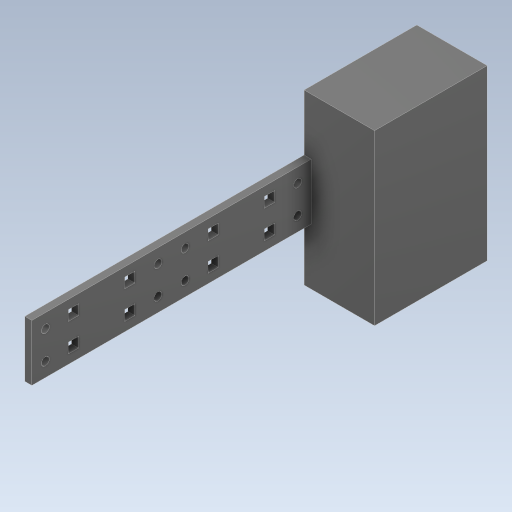
# Autodesk Inventor part: blocker
Saved by Autodesk Inventor 2024 (Build 280153000, 153)
## iProperties
Created: 2024-11-10
Part Number: blocker
Material: ABS Plastic
Document SubType Name: Modeling
Designer: Oscar
Density: 1.06 g/cm^3
Appearance: Smooth - Black
Author: Oscar
Autodesk Inventor part; units mm, degrees
ref_plane "YZ Plane" through (0, 0, 0) normal (1, 0, 0) x (0, 1, 0)
ref_plane "XZ Plane" through (0, 0, 0) normal (0, 1, 0) x (-1, 0, 0)
ref_plane "XY Plane" through (0, 0, 0) normal (0, 0, 1) x (1, 0, 0)
sketch "Sketch1" plane through (0, 0, 0) normal (1, 0, 0) x (0, 1, 0)
  line L0 (0, 0) -> (25.4, 0)
  line L1 (25.4, 0) -> (25.4, -126)
  line L2 (25.4, -126) -> (0, -126)
  line L3 (0, -126) -> (0, 0)
  line L4 (50.8, -126) -> (-25.4, -126)
  line L5 (-25.4, -126) -> (-25.4, -176.8)
  line L6 (-25.4, -176.8) -> (50.8, -176.8)
  line L7 (50.8, -176.8) -> (50.8, -126)
  line L8 (8.6614, -41.8886) -> (4.0386, -41.8886)
  line L9 (4.0386, -41.8886) -> (4.0386, -46.5114)
  line L10 (4.0386, -46.5114) -> (8.6614, -46.5114)
  line L11 (8.6614, -46.5114) -> (8.6614, -41.8886)
  line L12 (8.6614, -16.4886) -> (4.0386, -16.4886)
  line L13 (4.0386, -16.4886) -> (4.0386, -21.1114)
  line L14 (4.0386, -21.1114) -> (8.6614, -21.1114)
  line L15 (8.6614, -21.1114) -> (8.6614, -16.4886)
  line L16 (21.3614, -41.8886) -> (16.7386, -41.8886)
  line L17 (16.7386, -41.8886) -> (16.7386, -46.5114)
  line L18 (16.7386, -46.5114) -> (21.3614, -46.5114)
  line L19 (21.3614, -46.5114) -> (21.3614, -41.8886)
  line L20 (21.3614, -16.4886) -> (16.7386, -16.4886)
  line L21 (16.7386, -16.4886) -> (16.7386, -21.1114)
  line L22 (16.7386, -21.1114) -> (21.3614, -21.1114)
  line L23 (21.3614, -21.1114) -> (21.3614, -16.4886)
  line L24 (25.4, -63) -> (0, -63) construction
  line L25 (8.6614, -84.1114) -> (4.0386, -84.1114)
  line L26 (4.0386, -84.1114) -> (4.0386, -79.4886)
  line L27 (4.0386, -79.4886) -> (8.6614, -79.4886)
  line L28 (8.6614, -79.4886) -> (8.6614, -84.1114)
  line L29 (8.6614, -109.5114) -> (4.0386, -109.5114)
  line L30 (4.0386, -109.5114) -> (4.0386, -104.8886)
  line L31 (4.0386, -104.8886) -> (8.6614, -104.8886)
  line L32 (8.6614, -104.8886) -> (8.6614, -109.5114)
  line L33 (21.3614, -84.1114) -> (16.7386, -84.1114)
  line L34 (16.7386, -84.1114) -> (16.7386, -79.4886)
  line L35 (16.7386, -79.4886) -> (21.3614, -79.4886)
  line L36 (21.3614, -79.4886) -> (21.3614, -84.1114)
  line L37 (21.3614, -109.5114) -> (16.7386, -109.5114)
  line L38 (16.7386, -109.5114) -> (16.7386, -104.8886)
  line L39 (16.7386, -104.8886) -> (21.3614, -104.8886)
  line L40 (21.3614, -104.8886) -> (21.3614, -109.5114)
  circle A0 centre (19.05, -6.1) radius 1.8288
  circle A1 centre (6.35, -6.1) radius 1.8288
  circle A2 centre (19.05, -56.9) radius 1.8288
  circle A3 centre (6.35, -56.9) radius 1.8288
  circle A4 centre (19.05, -69.1) radius 1.8288
  circle A5 centre (6.35, -69.1) radius 1.8288
  circle A6 centre (19.05, -119.9) radius 1.8288
  circle A7 centre (6.35, -119.9) radius 1.8288
  point P0 (4.0386, -44.2)
  point P1 (4.0386, -18.8)
  point P2 (16.7386, -44.2)
  point P3 (16.7386, -18.8)
  point P4 (19.05, -21.1114)
  point P5 (6.35, -46.5114)
  point P6 (19.05, -16.4886)
  point P7 (6.35, -16.4886)
  point P8 (4.0386, -81.8)
  point P9 (4.0386, -107.2)
  point P10 (16.7386, -81.8)
  point P11 (16.7386, -107.2)
  point P12 (19.05, -104.8886)
  point P13 (6.35, -79.4886)
  point P14 (19.05, -109.5114)
  point P15 (6.35, -109.5114)
  point P16 (19.05, -109.5114)
  point P17 (0, -126)
  dimension "d0" = 25.4
  dimension "d1" = 126
  dimension "d2" = 76.2
  dimension "d3" = 50.8
  dimension "d4" = 25.4
  dimension "d5" = 4.6228
  dimension "d6" = 4.6228
  dimension "d13" = 25.4
  dimension "d14" = 25.4
  dimension "d16" = 12.7
  dimension "d17" = 6.35
  dimension "d19" = 18.8
  dimension "d20" = 3.6576
  dimension "d21" = 6.1
  dimension "d23" = 6.1
  dimension "d24" = 6.1
  dimension "d25" = 6.1
  constraints: 82 end point, 24 symmetric about line, 12 parallel, 11 midpoint, 10 vertical alignment, 8 centre point, 7 equal radius, 6 equal length, 6 horizontal, 6 perpendicular, 5 horizontal alignment, 1 point on line
  measures "d0" distance of L1.end L2.end
  measures "d1" distance of L0.end L1.end
  measures "d2" distance of L6.end L5.end
  measures "d3" distance of L5.end L4.end
  measures "d4" distance between parallel lines of L3 L5
  measures "d5" distance of L10.end L9.end
  measures "d6" distance of L9.end L8.end
  measures "d13" distance of point (4.039, -44.2) point (4.039, -18.8)
  measures "d14" distance of point (16.739, -44.2) point (16.739, -18.8)
  measures "d16" distance of point (19.05, -16.489) point (6.35, -16.489)
  measures "d17" distance from line of point (6.35, -16.489) L3
  measures "d19" distance from line of L0 point (16.739, -18.8)
  measures "d20" diameter of A0
  measures "d21" distance from line of L0 A0.centre
  measures "d23" distance from line of L24 A2.centre
  measures "d24" distance from line of L24 A4.centre
  measures "d25" distance from line of L2 A6.centre
extrude "Extrusion1" add sketch "Sketch1" along normal blind 3.175
sketch "Sketch2" plane through (3.175, 0, 0) normal (1, 0, 0) x (0, 0, -1)
  line L0 (126, 50.8) -> (126, 25.4) projected
  line L1 (176.8, -25.4) -> (176.8, 50.8) projected
  line L2 (126, 50.8) -> (176.8, 50.8)
  line L3 (176.8, 50.8) -> (176.8, -25.4)
  line L4 (176.8, -25.4) -> (126, -25.4)
  line L5 (126, -25.4) -> (126, 50.8)
  point P0 (0, 0)
  constraints: 8 end point, 2 parallel, 1 horizontal, 1 perpendicular
extrude "Extrusion2" add sketch "Sketch2" along normal blind 28.575
body "Solid1"
